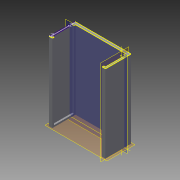
# Autodesk Inventor part: kontroller2
Saved by Autodesk Inventor 2015 (Build 190159000, 159)
## iProperties
Created: 2015-12-13
Part Number: kontroller2
Material: Generic
Document SubType Name: Modeling
Designer: abberik
Density: 1 g/cm^3
Appearance: Default
Author: abberik
Autodesk Inventor part; units mm, degrees
sketch "Sketch1" plane through (0, 0, 0) normal (0, 0, 1) x (1, 0, 0)
  line L0 (0, 2.868) -> (2, 2.868)
  line L1 (2, 2.868) -> (2, -21.132)
  line L2 (2, -21.132) -> (0, -21.132)
  line L3 (0, -21.132) -> (0, 2.868)
  line L4 (4, -23.132) -> (4, 4.868)
  line L5 (4, 4.868) -> (0, 4.868)
  line L6 (0, -23.132) -> (4, -23.132)
  line L7 (0, 2.868) -> (0, 4.868)
  line L8 (0, -23.132) -> (0, -21.132)
  line L9 (-30, 5.364) -> (-30, -29.5729)
  line L10 (-60, 2.868) -> (-62, 2.868)
  line L11 (-62, 2.868) -> (-62, -21.132)
  line L12 (-62, -21.132) -> (-60, -21.132)
  line L13 (-60, -21.132) -> (-60, 2.868)
  line L14 (-64, -23.132) -> (-64, 4.868)
  line L15 (-64, 4.868) -> (-60, 4.868)
  line L16 (-60, -23.132) -> (-64, -23.132)
  line L17 (-60, 2.868) -> (-60, 4.868)
  line L18 (-60, -23.132) -> (-60, -21.132)
  point P0 (0, 0)
  point P1 (-60, 0)
  dimension "d0" = 2
  dimension "d1" = 24
  dimension "d2" = 2
  dimension "d3" = 32
  constraints: 38 end point, 9 symmetric about line, 4 equal length, 3 perpendicular, 2 point on line, 1 horizontal, 1 vertical
  measures "d0" distance of L1.end L2.end
  measures "d1" distance of L0.end L1.end
  measures "d2" distance between parallel lines of L1 L4
  measures "d3" distance between parallel lines of L1 L9
extrude "Extrusion1" add sketch "Sketch1" along normal blind 94.2 contours L7 L5 L4 L6 L8 L2 L1 L0 | L10 L11 L12 L18 L16 L14 L15 L17
sketch "Sketch3" plane through (-64, 4.868, 0) normal (0, 1, 0) x (1, 0, 0)
  line L0 (4, 0) -> (0, 0) projected
  line L1 (0, 0) -> (0, -94.2) projected
  line L2 (4, -94.2) -> (0, -94.2) projected
  line L3 (4, 0) -> (4, -94.2) projected
  line L4 (68, 0) -> (64, 0) projected
  line L5 (64, 0) -> (64, -94.2) projected
  line L6 (68, -94.2) -> (64, -94.2) projected
  line L7 (68, 0) -> (68, -94.2) projected
  line L8 (0, 0) -> (68, 0)
  line L9 (68, 0) -> (68, -94.2)
  line L10 (68, -94.2) -> (0, -94.2)
  line L11 (0, -94.2) -> (0, 0)
  constraints: 8 end point, 2 parallel, 1 horizontal, 1 perpendicular
extrude "Extrusion2" add sketch "Sketch3" along normal blind 3
sketch "Sketch4" plane through (0, 0, 0) normal (0, 0, -1) x (-1, 0, 0)
  line L0 (0, 2.868) -> (-2, 2.868) projected
  line L1 (0, 4.868) -> (0, 2.868) projected
  line L2 (0, 4.868) -> (60, 4.868) projected
  line L3 (60, 2.868) -> (60, 4.868) projected
  line L4 (62, 2.868) -> (60, 2.868) projected
  line L5 (62, -21.132) -> (62, 2.868) projected
  line L6 (60, -21.132) -> (62, -21.132) projected
  line L7 (60, -23.132) -> (60, -21.132) projected
  line L8 (64, -23.132) -> (60, -23.132) projected
  line L9 (64, -23.132) -> (64, 7.868) projected
  line L10 (-4, 7.868) -> (64, 7.868) projected
  line L11 (-4, -23.132) -> (-4, 7.868) projected
  line L12 (0, -23.132) -> (-4, -23.132) projected
  line L13 (0, -21.132) -> (0, -23.132) projected
  line L14 (-2, -21.132) -> (0, -21.132) projected
  line L15 (-2, 2.868) -> (-2, -21.132) projected
  line L16 (-4, 7.868) -> (64, 7.868)
  line L17 (64, 7.868) -> (64, -23.132)
  line L18 (64, -23.132) -> (-4, -23.132)
  line L19 (-4, -23.132) -> (-4, 7.868)
  line L20 (0, -23.132) -> (0, 4.868)
  line L21 (0, 4.868) -> (60, 4.868)
  line L22 (60, -23.132) -> (60, 4.868)
  line L23 (60, -23.132) -> (60, -21.132) projected
  point P0 (0, 0)
  constraints: 14 end point, 2 parallel, 2 perpendicular, 1 collinear, 1 horizontal, 1 vertical
extrude "Extrusion3" add sketch "Sketch4" against normal blind 2 contours L20 L14 L15 L0 | L0 L15 L14 L13 L12 L11 L10 L9 L8 L7 L6 L5 L4 L3 L2 L1 | L4 L5 L6 L22
sketch "Sketch5" plane through (0, 0, 94.2) normal (0, 0, 1) x (1, 0, 0)
  line L0 (0, 2.868) -> (2, 2.868) projected
  line L1 (2, 2.868) -> (2, -21.132) projected
  line L2 (2, -21.132) -> (0, -21.132) projected
  line L3 (0, -21.132) -> (0, -23.132) projected
  line L4 (0, -23.132) -> (4, -23.132) projected
  line L5 (4, -23.132) -> (4, 7.868) projected
  line L6 (-64, 7.868) -> (4, 7.868) projected
  line L7 (-64, -23.132) -> (-64, 7.868) projected
  line L8 (-64, -23.132) -> (-60, -23.132) projected
  line L9 (-60, -23.132) -> (-60, -21.132) projected
  line L10 (-60, -21.132) -> (-62, -21.132) projected
  line L11 (-62, -21.132) -> (-62, 2.868) projected
  line L12 (-62, 2.868) -> (-60, 2.868) projected
  line L13 (-60, 2.868) -> (-60, 4.868) projected
  line L14 (-60, 4.868) -> (0, 4.868) projected
  line L15 (0, 4.868) -> (0, 2.868) projected
  line L16 (-62, 2.868) -> (-62, 0.868)
  line L17 (-62, -21.132) -> (-62, 2.868) projected
  line L18 (-62, 0.868) -> (-64, 0.868)
  line L19 (-62, -21.132) -> (-62, -19.132)
  line L20 (-62, -19.132) -> (-64, -19.132)
  line L21 (-64, -23.132) -> (-64, 7.868) projected
  line L22 (-64, -19.132) -> (-64, -23.132)
  line L23 (-64, 0.868) -> (-64, 7.868)
  line L24 (-64, 0.868) -> (-64, -19.132)
  line L25 (-62, -19.132) -> (-62, 0.868)
  line L26 (-62, -19.132) -> (-64, -19.132)
  line L27 (-64, 0.868) -> (-64, -19.132)
  line L28 (-62, -19.132) -> (-62, 0.868)
  line L29 (-62, 0.868) -> (-64, 0.868)
  line L30 (-64, 0.868) -> (-62, 0.868)
  line L31 (-62, 0.868) -> (-62, -21.132)
  line L32 (-62, -21.132) -> (-64, -21.132)
  line L33 (-64, -21.132) -> (-64, 0.868)
  point P0 (0, 0)
  dimension "d10" = 2
  dimension "d11" = 2
  constraints: 32 end point, 7 collinear, 4 point on line, 3 perpendicular, 2 horizontal, 2 parallel
  measures "d10" distance of L11.end L16.end
  measures "d11" distance of L10.end L19.end
body "Solid1"
